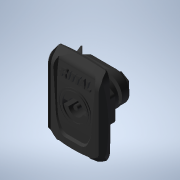
# Autodesk Inventor part: 1301.000_5_(1)
Saved by Autodesk Inventor 2021 (Build 250183000, 183)
## iProperties
Created: 2025-05-02
Part Number: 1301.000_5_(1)
Material: Generic
Catalog Web Link: www.cadenas.de
Description: Vorreibeverschluss EB Edelstahl 2.0-Vorreibeverschluss EB Edelstahl 2.0
Vendor: RITTAL
Document SubType Name: Modeling
Designer: psAdmin
Manufacturer: RITTAL
Mass: 18.9743 g
Surface Area: 89.9901 cm^2
Volume: 18.9743 cm^3
Density: 1 g/cm^3
Appearance: PSOLRGB-175-175-175
Category: PARTsolutions
Company: RITTAL
Title: 1301.000_5
Author: Cadenas PARTsolutions
Comments: Vorreibeverschluss EB Edelstahl 2.0
PSOL_IDENT_0: {$CADENAS_DATA/23d-libs/rittal/schaltschranksys/edelstahl/kleingehause/parts_eb_edel_2_0/vorreibever
PSOL_IDENT_1: schluss_kx_eb_edel_new.prj},205 {VTYP=3D},{NB=1301.000_5_(1)},{LINA=1301.000_5},{NN=Vorreibeverschlu
PSOL_IDENT_2: ss EB Edelstahl 2.0},{DATE=28.04.2025 21:10:48},{GEOMDATE=11.04.2025 11:21:29},{VERSION=},{LINEID=80
PSOL_IDENT_3: },{WBVAR=DETAIL},{WBNUMERIC=DETAIL}  {NB=1301.000_5_(1)},{LINA=1301.000_5},{KT=DUMMY},{BEST=1301.000
PSOL_IDENT_4: },{DETAIL=1},{GEW=3,889},{VERS=2},{CNSETIM80=EC000261},{CNSETIM90=EC000261},{CNSECLASS60=27-18-01-01
PSOL_IDENT_5: },{CNSECLASS80=27-18-01-01},{UNSPSC=31-26-15-02}
NB: 1301.000_5_(1)
NN: Vorreibeverschluss EB Edelstahl 2.0
NT: Vorreibeverschluss EB Edelstahl 2.0
NBSYN: $BEST._5_($DETAIL.)
LINA: 1301.000_5
CATALOG: Rittal
BEST: 1301.000
DETAIL: hoch
GEW: 3,889
VERS: 2
CNSETIM80: EC000261
CNSETIM90: EC000261
CNSECLASS60: 27-18-01-01
CNSECLASS80: 27-18-01-01
UNSPSC: 31-26-15-02
SUPPLIER: RITTAL
ARTICLENO: 1301.000_5_(1)
BOMINFO: 1301.000_5
CREATOR: CADENAS GmbH
Autodesk Inventor part; units mm, degrees
ref_plane "YZ Plane" through (0, 0, 0) normal (1, 0, 0) x (0, 1, 0)
ref_plane "XZ Plane" through (0, 0, 0) normal (0, 1, 0) x (-1, 0, 0)
ref_plane "XY Plane" through (0, 0, 0) normal (0, 0, 1) x (1, 0, 0)
sketch "Sketch_6" plane through (0, 0, 0) normal (0, -1, 0) x (1, 0, 0)
  line L0 (-17.65, 1.3) -> (-17.65, 0)
  line L1 (-17.65, 0) -> (17.65, 0)
  line L2 (17.65, 0) -> (17.65, 1.3)
  line L3 (17.65, 1.3) -> (16.6449, 7)
  line L4 (16.6449, 7) -> (-16.6449, 7)
  line L5 (-16.6449, 7) -> (-17.65, 1.3)
  constraints: 12 end point
extrude "Extrusion1" add sketch "Sketch_6" along normal mid plane 55.1
sketch "Sketch_1" plane through (0, 0, 7) normal (0, 0, 1) x (1, 0, 0)
  line L0 (-15.2906, 36.1) -> (-14.1918, 16.1075)
  arc A0 (-14.1918, 16.1075) -> (-14.0539, 14.1707) centre (45.7178, 19.4001) ccw
  line L1 (-14.0539, 14.1707) -> (-12.1282, -7.84)
  arc A1 (-12.1282, -7.84) -> (-10.69, -13.2074) centre (3.8109, -6.4455) ccw
  line L2 (-10.69, -13.2074) -> (-9.7308, -15.2644)
  arc A2 (-9.7308, -15.2644) -> (-4.7461, -18.44) centre (-4.7461, -12.94) ccw
  line L3 (-4.7461, -18.44) -> (4.7461, -18.44)
  arc A3 (4.7461, -18.44) -> (9.7308, -15.2644) centre (4.7461, -12.94) ccw
  line L4 (9.7308, -15.2644) -> (10.69, -13.2074)
  arc A4 (10.69, -13.2074) -> (12.1282, -7.84) centre (-3.8109, -6.4455) ccw
  line L5 (12.1282, -7.84) -> (14.0539, 14.1707)
  arc A5 (14.0539, 14.1707) -> (14.1918, 16.1075) centre (-45.7178, 19.4001) ccw
  line L6 (14.1918, 16.1075) -> (15.2906, 36.1)
  line L7 (15.2906, 36.1) -> (-15.2906, 36.1)
  constraints: 16 end point, 12 point on circle, 6 centre point
extrude "Extrusion2" cut sketch "Sketch_1" against normal blind 5.7 draft -42
sketch "Sketch_43" plane through (0, 0, 0) normal (0, 0, 1) x (1, 0, 0)
  line L0 (-10.3, 19.67) -> (-10.3, 13.67)
  line L1 (-10.3, 13.67) -> (10.6, 13.67)
  line L2 (10.6, 13.67) -> (10.6, 19.67)
  line L3 (10.6, 19.67) -> (-10.3, 19.67)
  constraints: 8 end point
extrude "Extrusion3" add sketch "Sketch_43" along normal blind 6
sketch "Sketch_44" plane through (0, 0, 6) normal (0, 0, 1) x (1, 0, 0)
  line L0 (-10.3, 19.67) -> (-10.3, 13.67)
  line L1 (-10.3, 13.67) -> (10.6, 13.67)
  line L2 (10.6, 13.67) -> (10.6, 19.67)
  line L3 (10.6, 19.67) -> (-10.3, 19.67)
  line L4 (6.723, 14.166) -> (10.118, 14.163)
  line L5 (10.118, 14.163) -> (10.118, 15.294)
  line L6 (10.118, 15.294) -> (8.245, 15.296)
  line L7 (8.245, 15.296) -> (9.308, 19.31)
  line L8 (9.308, 19.31) -> (8.088, 19.312)
  line L9 (8.088, 19.312) -> (6.723, 14.166)
  line L10 (1.861, 14.171) -> (3.212, 14.17)
  line L11 (3.212, 14.17) -> (3.783, 15.104)
  line L12 (3.783, 15.104) -> (5.252, 15.102)
  line L13 (5.252, 15.102) -> (5.324, 14.167)
  line L14 (5.324, 14.167) -> (6.584, 14.167)
  line L15 (6.584, 14.167) -> (6.063, 19.317)
  line L16 (6.063, 19.317) -> (5.132, 19.318)
  line L17 (5.132, 19.318) -> (1.861, 14.171)
  line L18 (0.388, 14.17) -> (1.615, 14.171)
  line L19 (1.615, 14.171) -> (2.697, 18.191)
  line L20 (2.697, 18.191) -> (3.434, 18.191)
  line L21 (3.434, 18.191) -> (3.738, 19.323)
  line L22 (3.738, 19.323) -> (0.875, 19.322)
  line L23 (0.875, 19.322) -> (0.57, 18.19)
  line L24 (0.57, 18.19) -> (1.472, 18.19)
  line L25 (1.472, 18.19) -> (0.388, 14.17)
  line L26 (-2.753, 14.17) -> (-1.526, 14.171)
  line L27 (-1.526, 14.171) -> (-0.444, 18.191)
  line L28 (-0.444, 18.191) -> (0.292, 18.191)
  line L29 (0.292, 18.191) -> (0.596, 19.323)
  line L30 (0.596, 19.323) -> (-2.267, 19.322)
  line L31 (-2.267, 19.322) -> (-2.571, 18.19)
  line L32 (-2.571, 18.19) -> (-1.669, 18.19)
  line L33 (-1.669, 18.19) -> (-2.753, 14.17)
  line L34 (-5.308, 14.168) -> (-4.083, 14.169)
  line L35 (-4.083, 14.169) -> (-2.693, 19.322)
  line L36 (-2.693, 19.322) -> (-3.916, 19.32)
  line L37 (-3.916, 19.32) -> (-5.308, 14.168)
  line L38 (-9.987, 17.217) -> (-9.987, 16.139)
  line L39 (-9.987, 16.139) -> (-9.151, 16.14)
  line L40 (-9.151, 16.14) -> (-9.687, 14.161)
  line L41 (-9.687, 14.161) -> (-8.467, 14.163)
  line L42 (-8.467, 14.163) -> (-7.936, 16.124)
  line L43 (-7.936, 16.124) -> (-7.443, 16.125)
  line L44 (-7.443, 16.125) -> (-6.993, 14.165)
  line L45 (-6.993, 14.165) -> (-5.649, 14.166)
  line L46 (-5.649, 14.166) -> (-6.179, 16.315)
  arc A0 (-6.179, 16.315) -> (-5.144, 17.102) centre (-6.971, 18.4306) ccw
  arc A1 (-5.144, 17.102) -> (-5.144, 18.833) centre (-6.4742, 17.9675) ccw
  arc A2 (-5.144, 18.833) -> (-6.3, 19.316) centre (-6.2287, 17.8617) ccw
  line L47 (-6.3, 19.316) -> (-8.293, 19.312)
  line L48 (-8.293, 19.312) -> (-8.86, 17.218)
  line L49 (-8.86, 17.218) -> (-9.987, 17.217)
  constraints: 100 end point, 6 point on circle, 3 centre point
extrude "Extrusion4" cut sketch "Sketch_44" against normal blind 2
sketch "Sketch_46" plane through (0, 0, 6) normal (0, 0, 1) x (1, 0, 0)
  line L0 (-7.614, 17.216) -> (-6.897, 17.216)
  arc A0 (-6.897, 17.216) -> (-6.428, 17.356) centre (-6.8725, 17.9896) ccw
  arc A1 (-6.428, 17.356) -> (-6.13, 17.839) centre (-6.9274, 17.9975) ccw
  arc A2 (-6.13, 17.839) -> (-6.192, 18.075) centre (-6.3798, 17.8995) ccw
  arc A3 (-6.192, 18.075) -> (-6.457, 18.174) centre (-6.4312, 17.839) ccw
  line L1 (-6.457, 18.174) -> (-7.356, 18.174)
  line L2 (-7.356, 18.174) -> (-7.614, 17.216)
  constraints: 8 point on circle, 6 end point, 4 centre point
extrude "Extrusion5" cut sketch "Sketch_46" against normal blind 2
sketch "Sketch_47" plane through (0, 0, 6) normal (0, 0, 1) x (1, 0, 0)
  line L0 (4.4417, 16.1815) -> (5.2647, 16.1805)
  line L1 (5.2647, 16.1805) -> (5.2027, 17.4445)
  line L2 (5.2027, 17.4445) -> (4.4417, 16.1815)
  constraints: 6 end point
extrude "Extrusion6" cut sketch "Sketch_47" against normal blind 2
sketch "Sketch_2" plane through (0, 0, 7) normal (1, 0, 0) x (0, 0, -1)
  arc A0 (2.6402, 21.4) -> (1.4014, -20) centre (279.4, -7.6) ccw
  arc A1 (1.4014, -20) -> (4.1718, -25.8207) centre (8.9014, -20) ccw
  line L0 (4.1718, -25.8207) -> (6.3, -27.55)
  line L1 (6.3, -27.55) -> (6.3, 27.55)
  line L2 (6.3, 27.55) -> (5.7, 27.55)
  line L3 (5.7, 27.55) -> (3.5376, 24.258)
  arc A2 (3.5376, 24.258) -> (2.6402, 21.4) centre (7.6402, 21.4) ccw
  constraints: 8 end point, 6 point on circle, 3 centre point
extrude "Extrusion7" add sketch "Sketch_2" along normal mid plane 32
sketch "Sketch_5" plane through (0, 0, 0) normal (0, 0, 1) x (1, 0, 0)
  line L0 (-40, -50) -> (40, -50)
  line L1 (40, -50) -> (40, 50)
  line L2 (40, 50) -> (-40, 50)
  line L3 (-40, 50) -> (-40, -50)
  arc A0 (-17.177, 19.885) -> (-17.448, -18.485) centre (559.8053, -3.3761) ccw
  arc A1 (-17.448, -18.485) -> (-17.092, -21.203) centre (-6.801, -18.4728) ccw
  arc A2 (-17.092, -21.203) -> (-16.213, -23.36) centre (-4.8797, -17.484) ccw
  arc A3 (-16.213, -23.36) -> (-15.393, -24.9) centre (8.4697, -11.2056) ccw
  arc A4 (-15.393, -24.9) -> (-12.239, -26.766) centre (4.8714, 5.7533) ccw
  arc A5 (-12.239, -26.766) -> (-12.0566, -26.7175) centre (-13.4109, -21.9938) ccw
  arc A6 (-12.0566, -26.7175) -> (12.0566, -26.7175) centre (0, 72) ccw
  arc A7 (12.0566, -26.7175) -> (12.239, -26.766) centre (13.4109, -21.9938) ccw
  arc A8 (12.239, -26.766) -> (15.393, -24.9) centre (-4.8714, 5.7533) ccw
  arc A9 (15.393, -24.9) -> (16.213, -23.36) centre (-8.4697, -11.2056) ccw
  arc A10 (16.213, -23.36) -> (17.092, -21.203) centre (4.8797, -17.484) ccw
  arc A11 (17.092, -21.203) -> (17.448, -18.485) centre (6.801, -18.4728) ccw
  arc A12 (17.448, -18.485) -> (17.177, 19.885) centre (-559.8053, -3.3761) ccw
  arc A13 (17.177, 19.885) -> (16.263, 24.293) centre (6.3822, 19.9454) ccw
  arc A14 (16.263, 24.293) -> (15.412, 26.294) centre (-21.6414, 9.3542) ccw
  line L4 (15.412, 26.294) -> (14.58, 26.682)
  line L5 (14.58, 26.682) -> (14.2616, 26.6294)
  arc A15 (14.2616, 26.6294) -> (-14.2616, 26.6294) centre (0, -75.227) ccw
  line L6 (-14.2616, 26.6294) -> (-14.58, 26.682)
  line L7 (-14.58, 26.682) -> (-15.412, 26.294)
  arc A16 (-15.412, 26.294) -> (-16.263, 24.293) centre (21.6414, 9.3542) ccw
  arc A17 (-16.263, 24.293) -> (-17.177, 19.885) centre (-6.3822, 19.9454) ccw
  constraints: 36 point on circle, 18 centre point, 16 end point
extrude "Extrusion8" cut sketch "Sketch_5" along normal blind 20
sketch "Sketch_7" plane through (0, 27.55, 1.3) normal (0, -0.7660444, 0.6427876) x (1, 0, 0)
  line L0 (-38, -25) -> (-17.65, -25)
  line L1 (-17.65, -25) -> (-17.65, -1.5387)
  line L2 (-17.65, -1.5387) -> (-16.8432, -0.3865)
  arc A0 (-16.3432, -0.3049) -> (-16.8432, -0.3865) centre (0, -102) ccw
  line L3 (-16.3432, -0.3049) -> (-15.593, -1.1989)
  arc A1 (15.593, -1.1989) -> (-15.593, -1.1989) centre (0, -102) ccw
  line L4 (15.593, -1.1989) -> (16.3432, -0.3049)
  arc A2 (16.8432, -0.3865) -> (16.3432, -0.3049) centre (0, -102) ccw
  line L5 (16.8432, -0.3865) -> (17.65, -1.5387)
  line L6 (17.65, -1.5387) -> (17.65, -25)
  line L7 (17.65, -25) -> (35, -25)
  line L8 (35, -25) -> (35, 19)
  line L9 (35, 19) -> (-38, 19)
  line L10 (-38, 19) -> (-38, -25)
  constraints: 22 end point, 6 point on circle, 3 centre point
extrude "Extrusion9" cut sketch "Sketch_7" along normal blind 20
sketch "Sketch_8" plane through (0, 23.3368, 4.8353) normal (0, -0.7660444, 0.6427876) x (1, 0, 0)
  line L0 (50, -10) -> (-50, -10)
  line L1 (-38, -6) -> (-17.65, -6)
  line L2 (-17.65, -6) -> (-17.65, -1.5387)
  line L3 (-17.65, -1.5387) -> (-16.8432, -0.3865)
  arc A0 (-16.3432, -0.3049) -> (-16.8432, -0.3865) centre (0, -102) ccw
  line L4 (-16.3432, -0.3049) -> (-15.593, -1.1989)
  arc A1 (15.593, -1.1989) -> (-15.593, -1.1989) centre (0, -102) ccw
  line L5 (15.593, -1.1989) -> (16.3432, -0.3049)
  arc A2 (16.8432, -0.3865) -> (16.3432, -0.3049) centre (0, -102) ccw
  line L6 (16.8432, -0.3865) -> (17.65, -1.5387)
  line L7 (17.65, -1.5387) -> (17.65, -6)
  line L8 (17.65, -6) -> (35, -6)
  line L9 (35, -6) -> (35, 19)
  line L10 (35, 19) -> (-38, 19)
  line L11 (-38, 19) -> (-38, -6)
  constraints: 24 end point, 6 point on circle, 3 centre point
revolve "Revolution1" cut sketch "Sketch_8" angle 40 about axis through (50, 16.9089, -2.8251) along (1, 0, 0)
sketch "Sketch_9" plane through (0, 16.9089, 7.1749) normal (0, -1, 0) x (1, 0, 0)
  line L0 (-38, -6) -> (-17.65, -6)
  line L1 (-17.65, -6) -> (-17.65, -1.5387)
  line L2 (-17.65, -1.5387) -> (-16.8432, -0.3865)
  arc A0 (-16.3432, -0.3049) -> (-16.8432, -0.3865) centre (0, -102) ccw
  line L3 (-16.3432, -0.3049) -> (-15.593, -1.1989)
  arc A1 (15.593, -1.1989) -> (-15.593, -1.1989) centre (0, -102) ccw
  line L4 (15.593, -1.1989) -> (16.3432, -0.3049)
  arc A2 (16.8432, -0.3865) -> (16.3432, -0.3049) centre (0, -102) ccw
  line L5 (16.8432, -0.3865) -> (17.65, -1.5387)
  line L6 (17.65, -1.5387) -> (17.65, -6)
  line L7 (17.65, -6) -> (35, -6)
  line L8 (35, -6) -> (35, 19)
  line L9 (35, 19) -> (-38, 19)
  line L10 (-38, 19) -> (-38, -6)
  constraints: 22 end point, 6 point on circle, 3 centre point
extrude "Extrusion10" cut sketch "Sketch_9" along normal blind 43
sketch "Sketch_11" plane through (0, -27.55, 1.3) normal (0, 0.6427876, 0.7660444) x (1, 0, 0)
  line L0 (-41.5728, -20.604) -> (38.4272, -20.604)
  line L1 (38.4272, -20.604) -> (38.4272, 19.396)
  line L2 (38.4272, 19.396) -> (17.65, 19.396)
  line L3 (17.65, 19.396) -> (17.65, 4.3312)
  arc A0 (11.0304, 0.25) -> (17.65, 4.3312) centre (0, 25.55) ccw
  line L4 (11.0304, 0.25) -> (10.2426, 0.5367)
  arc A1 (-10.2426, 0.5367) -> (10.2426, 0.5367) centre (0, 98) ccw
  line L5 (-10.2426, 0.5367) -> (-11.0304, 0.25)
  arc A2 (-17.65, 4.3312) -> (-11.0304, 0.25) centre (0, 25.55) ccw
  line L6 (-17.65, 4.3312) -> (-17.65, 19.396)
  line L7 (-17.65, 19.396) -> (-41.5728, 19.396)
  line L8 (-41.5728, 19.396) -> (-41.5728, -20.604)
  constraints: 18 end point, 6 point on circle, 3 centre point
extrude "Extrusion11" cut sketch "Sketch_11" along normal blind 40
sketch "Sketch_17" plane through (0, 0, 0) normal (0, 1, 0) x (-1, 0, 0)
  line L0 (0, 0) -> (0, -21.4)
  line L1 (0, -19.9) -> (-6.95, -19.9)
  arc A0 (-6.95, -19.9) -> (-7.25, -20.2) centre (-6.95, -20.2) ccw
  line L2 (-7.25, -20.2) -> (-7.25, -20.6)
  arc A1 (-8.05, -21.4) -> (-7.25, -20.6) centre (-8.05, -20.6) ccw
  line L3 (-8.05, -21.4) -> (-8.5, -21.4)
  arc A2 (-9.5, -20.4) -> (-8.5, -21.4) centre (-8.5, -20.4) ccw
  line L4 (-9.5, -20.4) -> (-9.5, -15.9)
  line L5 (-9.5, -15.9) -> (-4.95, -15.9)
  line L6 (-4.95, -15.9) -> (-4.95, -15.8)
  line L7 (-4.95, -15.8) -> (-9.75, -15.8)
  line L8 (-9.75, -15.8) -> (-9.75, -9.7)
  line L9 (-9.75, -9.7) -> (-9.773, -9.7)
  line L10 (-9.773, -9.7) -> (-11, -8.473)
  line L11 (-11, -8.473) -> (-11, -2.5)
  line L12 (-11, -2.5) -> (-10.125, -2.5)
  line L13 (-10.125, -2.5) -> (-10.125, 0)
  line L14 (-10.125, 0) -> (0, 0)
  line L15 (0, 0) -> (0, -19.9)
  constraints: 32 end point, 6 point on circle, 3 centre point
revolve "Revolution2" add sketch "Sketch_17" angle 360 about axis through (0, 0, 0) along (0, 0, 1)
thread "Thread1" size "M22x2" class "6g" standard "ISO Metric profile" full length
sketch "Sketch_19" plane through (0, 0, 0) normal (0, 0, 1) x (1, 0, 0)
  line L0 (-11.1, 11.1) -> (-11.1, -11.1)
  line L1 (-11.1, -11.1) -> (11.1, -11.1)
  line L2 (11.1, -11.1) -> (11.1, 11.1)
  line L3 (11.1, 11.1) -> (-11.1, 11.1)
  line L4 (-10, -10) -> (10, -10)
  line L5 (10, -10) -> (10, 10)
  line L6 (10, 10) -> (-10, 10)
  line L7 (-10, 10) -> (-10, -10)
  constraints: 16 end point
extrude "Extrusion12" cut sketch "Sketch_19" against normal blind 10
sketch "Sketch_20" plane through (0, 0, 0) normal (0, 0, 1) x (1, 0, 0)
  arc A0 (-14.7, -10.2) -> (-10.2, -14.7) centre (-10.2, -10.2) ccw
  line L0 (-10.2, -14.7) -> (10.2, -14.7)
  arc A1 (10.2, -14.7) -> (14.7, -10.2) centre (10.2, -10.2) ccw
  line L1 (14.7, -10.2) -> (14.7, 10.2)
  arc A2 (14.7, 10.2) -> (10.2, 14.7) centre (10.2, 10.2) ccw
  line L2 (10.2, 14.7) -> (-10.2, 14.7)
  arc A3 (-10.2, 14.7) -> (-14.7, 10.2) centre (-10.2, 10.2) ccw
  line L3 (-14.7, 10.2) -> (-14.7, -10.2)
  constraints: 8 end point, 8 point on circle, 4 centre point
extrude "Extrusion13" add sketch "Sketch_20" against normal blind 1.07
sketch "Sketch_18" plane through (0, 0, -15.9) normal (0, 0, 1) x (1, 0, 0)
  line L0 (-10, 10.2) -> (-10, -2.8)
  line L1 (-10, -2.8) -> (-4.082, -2.8)
  arc A0 (4.082, -2.8) -> (-4.082, -2.8) centre (0, 0) ccw
  line L2 (4.082, -2.8) -> (10, -2.8)
  line L3 (10, -2.8) -> (10, 10.2)
  line L4 (10, 10.2) -> (-10, 10.2)
  constraints: 10 end point, 2 point on circle, 1 centre point
extrude "Extrusion14" cut sketch "Sketch_18" along normal blind 2.4
sketch "Sketch_21" plane through (0, 0, -15.9) normal (0, 0, 1) x (1, 0, 0)
  arc A0 (-5.5, 7.7942) -> (-5.5, -7.7942) centre (-1, 0) ccw
  line L0 (-5.5, -7.7942) -> (-4.75, -8.2272)
  arc A1 (-4.75, -8.2272) -> (-4.75, 8.2272) centre (0, 0) ccw
  line L1 (-4.75, 8.2272) -> (-5.5, 7.7942)
  constraints: 4 end point, 4 point on circle, 2 centre point
extrude "Extrusion15" add sketch "Sketch_21" against normal blind 4.5
sketch "Sketch_22" plane through (0, 0, -15.9) normal (0, 0, 1) x (1, 0, 0)
  arc A0 (-9.5534, 2.8) -> (-9.5534, -2.8) centre (-1, 0) ccw
  line L0 (-9.5534, -2.8) -> (0, -2.8)
  line L1 (0, -2.8) -> (0, 2.8)
  line L2 (0, 2.8) -> (-9.5534, 2.8)
  constraints: 6 end point, 2 point on circle, 1 centre point
extrude "Extrusion16" add sketch "Sketch_22" along normal blind 2.3
sketch "Sketch_23" plane through (0, 0, 0) normal (1, 0, 0) x (0, 1, 0)
  line L0 (6.5, -17.4) -> (-6.5, -17.4)
  line L1 (-6.5, -17.4) -> (-9.5, -18.7989)
  line L2 (-9.5, -18.7989) -> (-9.5, -20.4)
  arc A0 (-9.5, -20.4) -> (-8.5, -21.4) centre (-8.5, -20.4) ccw
  line L3 (-8.5, -21.4) -> (8.5, -21.4)
  arc A1 (8.5, -21.4) -> (9.5, -20.4) centre (8.5, -20.4) ccw
  line L4 (9.5, -20.4) -> (9.5, -18.7989)
  line L5 (9.5, -18.7989) -> (6.5, -17.4)
  constraints: 12 end point, 4 point on circle, 2 centre point
extrude "Extrusion17" add sketch "Sketch_23" against normal blind 20
sketch "Sketch_45" plane through (0, 0, 0) normal (0, 1, 0) x (-1, 0, 0)
  line L0 (28.466, -23.355) -> (23.0968, -17.9858)
  arc A0 (23.0968, -17.9858) -> (21.6826, -17.4) centre (21.6826, -19.4) ccw
  line L1 (21.6826, -17.4) -> (14.511, -17.4)
  line L2 (14.511, -17.4) -> (14.511, -21.4)
  line L3 (14.511, -21.4) -> (16.7433, -21.4)
  arc A1 (18.1575, -21.9858) -> (16.7433, -21.4) centre (16.7433, -23.4) ccw
  line L4 (18.1575, -21.9858) -> (21.3575, -25.1857)
  arc A2 (21.3575, -25.1857) -> (21.8057, -25.4445) centre (22.0646, -24.4786) ccw
  line L5 (21.8057, -25.4445) -> (24.853, -26.261)
  arc A3 (24.853, -26.261) -> (25.8189, -26.0022) centre (25.1118, -25.2951) ccw
  line L6 (25.8189, -26.0022) -> (28.466, -23.355)
  constraints: 14 end point, 8 point on circle, 4 centre point
extrude "Extrusion18" add sketch "Sketch_45" along normal mid plane 13.7
sketch "Sketch_24" plane through (-20.3897, 0, -15.2787) normal (-0.7071068, 0, -0.7071068) x (-0.7071068, 0, 0.7071068)
  line L0 (-4.0663, -9.85) -> (5, -9.85)
  line L1 (5, -9.85) -> (5, 9.85)
  line L2 (5, 9.85) -> (-4.0663, 9.85)
  line L3 (-4.0663, 9.85) -> (0, 3)
  line L4 (0, 3) -> (0, -3)
  line L5 (0, -3) -> (-4.0663, -9.85)
  constraints: 12 end point
extrude "Extrusion19" cut sketch "Sketch_24" along normal blind 13
sketch "Sketch_25" plane through (-20.319, 0, -19.592) normal (-0.7071068, 0, 0.7071068) x (0.7071068, 0, 0.7071068)
  line L0 (-21.047, 9.5) -> (-21.047, -9.5)
  line L1 (-21.047, -9.5) -> (2.078, -9.5)
  line L2 (2.078, -9.5) -> (2.078, -3.7)
  arc A0 (2.078, -3.7) -> (0.378, -2) centre (0.378, -3.7) ccw
  line L3 (0.378, -2) -> (-12.922, -2)
  line L4 (-12.922, -2) -> (-12.922, 2)
  line L5 (-12.922, 2) -> (0.378, 2)
  arc A1 (0.378, 2) -> (2.078, 3.7) centre (0.378, 3.7) ccw
  line L6 (2.078, 3.7) -> (2.078, 9.5)
  line L7 (2.078, 9.5) -> (-21.047, 9.5)
  constraints: 16 end point, 4 point on circle, 2 centre point
extrude "Extrusion20" cut sketch "Sketch_25" against normal blind 5
sketch "Sketch_26" plane through (-20.319, 0, -19.592) normal (-0.7071068, 0, 0.7071068) x (0.7071068, 0, 0.7071068)
  line L0 (-12.922, -10.85) -> (2.078, -10.85)
  line L1 (2.078, -10.85) -> (2.078, -6.85)
  line L2 (2.078, -6.85) -> (-12.922, -6.85)
  line L3 (-12.922, -6.85) -> (-12.922, -10.85)
  constraints: 8 end point
extrude "Extrusion21" cut sketch "Sketch_26" along normal blind 3
sketch "Sketch_27" plane through (-20.319, 0, -19.592) normal (-0.7071068, 0, 0.7071068) x (0.7071068, 0, 0.7071068)
  line L0 (-12.922, 10.85) -> (-12.922, 6.85)
  line L1 (-12.922, 6.85) -> (2.078, 6.85)
  line L2 (2.078, 6.85) -> (2.078, 10.85)
  line L3 (2.078, 10.85) -> (-12.922, 10.85)
  constraints: 8 end point
extrude "Extrusion22" cut sketch "Sketch_27" along normal blind 3
sketch "Sketch_28" plane through (-22.511, 0, -17.4) normal (1, 0, 0) x (0, 0, -1)
  line L0 (-3, 9.5) -> (-3, -9.5)
  line L1 (-3, -9.5) -> (1.3989, -9.5)
  line L2 (1.3989, -9.5) -> (0, -6.5)
  line L3 (0, -6.5) -> (0, 6.5)
  line L4 (0, 6.5) -> (1.3989, 9.5)
  line L5 (1.3989, 9.5) -> (-3, 9.5)
  constraints: 12 end point
extrude "Extrusion23" cut sketch "Sketch_28" along normal blind 8
sketch "Sketch_36" plane through (0, 0, 0) normal (0, 1, 0) x (-1, 0, 0)
  line L0 (0, 0) -> (0, -21.4)
  line L1 (0, -21.4) -> (-8.05, -21.4)
  arc A0 (-8.05, -21.4) -> (-7.25, -20.6) centre (-8.05, -20.6) ccw
  line L2 (-7.25, -20.6) -> (-7.25, -20.2)
  arc A1 (-6.95, -19.9) -> (-7.25, -20.2) centre (-6.95, -20.2) ccw
  line L3 (-6.95, -19.9) -> (0, -19.9)
  line L4 (0, -19.9) -> (0, -21.4)
  constraints: 10 end point, 4 point on circle, 2 centre point
revolve "Revolution3" cut sketch "Sketch_36" angle 360 about axis through (0, 0, 0) along (0, 0, 1)
sketch "Sketch_10" plane through (0, 0, 0) normal (0, 0, 1) x (1, 0, 0)
  circle A0 centre (0, 0) radius 9.05
  constraints: 1 centre point
extrude "Extrusion24" add sketch "Sketch_10" along normal blind 6
sketch "Sketch_12" plane through (0, 0, 6) normal (0, 0, 1) x (1, 0, 0)
  circle A0 centre (0, 0) radius 8
  constraints: 1 centre point
extrude "Extrusion25" cut sketch "Sketch_12" along normal mid plane 1.4
sketch "Sketch_16" plane through (0, 0, 0) normal (0, 0, 1) x (1, 0, 0)
  circle A0 centre (0, 0) radius 10.75
  circle A1 centre (0, 0) radius 10
  constraints: 2 centre point
extrude "Extrusion26" add sketch "Sketch_16" along normal blind 6
sketch "Sketch_13" plane through (0, 0, 5.3) normal (0, 0, 1) x (1, 0, 0)
  arc A0 (-7.8581, 1.5) -> (-7.8581, -1.5) centre (0, 0) ccw
  line L0 (-7.8581, -1.5) -> (-4.7697, -1.5)
  arc A1 (-4.7697, -1.5) -> (4.7697, -1.5) centre (0, 0) ccw
  line L1 (4.7697, -1.5) -> (7.8581, -1.5)
  arc A2 (7.8581, -1.5) -> (7.8581, 1.5) centre (0, 0) ccw
  line L2 (7.8581, 1.5) -> (4.7697, 1.5)
  arc A3 (4.7697, 1.5) -> (-4.7697, 1.5) centre (0, 0) ccw
  line L3 (-4.7697, 1.5) -> (-7.8581, 1.5)
  circle A4 centre (0, 0) radius 1.5
  constraints: 8 end point, 8 point on circle, 5 centre point
extrude "Extrusion27" cut sketch "Sketch_13" against normal blind 7.5
sketch "Sketch_14" plane through (0, 0, -19.9) normal (0, 0, 1) x (1, 0, 0)
  line L0 (-5, -2.8868) -> (0, -5.7735)
  line L1 (0, -5.7735) -> (5, -2.8868)
  line L2 (5, -2.8868) -> (5, 2.8868)
  line L3 (5, 2.8868) -> (0, 5.7735)
  line L4 (0, 5.7735) -> (-5, 2.8868)
  line L5 (-5, 2.8868) -> (-5, -2.8868)
  constraints: 12 end point
extrude "Extrusion28" add sketch "Sketch_14" against normal blind 5
sketch "Sketch_35" plane through (0, 0, 0) normal (0, 1, 0) x (-1, 0, 0)
  line L0 (0, -19.9) -> (0, -20.15)
  arc A0 (-6.75, -20.1497) -> (0, -20.8997) centre (-1.423, -2.956) ccw
  line L1 (-6.75, -20.1497) -> (-6.75, -19.9)
  line L2 (-6.75, -19.9) -> (0, -19.9)
  line L3 (0, -19.9) -> (0, -20.8997)
  constraints: 8 end point, 2 point on circle, 1 centre point
revolve "Revolution4" add sketch "Sketch_35" angle 360 about axis through (0, 0, -19.9) along (0, 0, 1)
sketch "Sketch_40" plane through (0, 0, 0) normal (1, 0, 0) x (0, 1, 0)
  line L0 (0, -7.4) -> (0, -2.6)
  line L1 (11.5, -2.6) -> (10.3, -3.2928)
  line L2 (10.3, -3.2928) -> (10.3, -6.7072)
  line L3 (10.3, -6.7072) -> (11.5, -7.4)
  line L4 (11.5, -7.4) -> (15.3, -7.4)
  line L5 (15.3, -7.4) -> (15.3, -2.6)
  line L6 (15.3, -2.6) -> (11.5, -2.6)
  constraints: 14 end point
revolve "Revolution5" add sketch "Sketch_40" angle 360 about axis through (0, 0, -7.4) along (0, 0, -1)
sketch "Sketch_41" plane through (0, 0, -7.4) normal (0, 0, 1) x (1, 0, 0)
  line L0 (-27, -27) -> (27, -27)
  line L1 (27, -27) -> (27, 27)
  line L2 (27, 27) -> (-27, 27)
  line L3 (-27, 27) -> (-27, -27)
  arc A0 (-13.5, -6.6395) -> (-12.5, -8.3716) centre (-11.5, -6.6395) ccw
  line L4 (-12.5, -8.3716) -> (-1, -15.0111)
  arc A1 (-1, -15.0111) -> (1, -15.0111) centre (0, -13.2791) ccw
  line L5 (1, -15.0111) -> (12.5, -8.3716)
  arc A2 (12.5, -8.3716) -> (13.5, -6.6395) centre (11.5, -6.6395) ccw
  line L6 (13.5, -6.6395) -> (13.5, 6.6395)
  arc A3 (13.5, 6.6395) -> (12.5, 8.3716) centre (11.5, 6.6395) ccw
  line L7 (12.5, 8.3716) -> (1, 15.0111)
  arc A4 (1, 15.0111) -> (-1, 15.0111) centre (0, 13.2791) ccw
  line L8 (-1, 15.0111) -> (-12.5, 8.3716)
  arc A5 (-12.5, 8.3716) -> (-13.5, 6.6395) centre (-11.5, 6.6395) ccw
  line L9 (-13.5, 6.6395) -> (-13.5, -6.6395)
  constraints: 20 end point, 12 point on circle, 6 centre point
extrude "Extrusion29" cut sketch "Sketch_41" along normal blind 4.8
sketch "Sketch_29" plane through (0, 0, -2.6) normal (0, 0, 1) x (1, 0, 0)
  arc A0 (-13.5, -6.6395) -> (-12.5, -8.3716) centre (-11.5, -6.6395) ccw
  line L0 (-12.5, -8.3716) -> (-9.8827, -9.8827)
  line L1 (-9.8827, -9.8827) -> (-9.5459, -9.5459)
  arc A1 (-13.04, -3.4941) -> (-9.5459, -9.5459) centre (0, 0) ccw
  line L2 (-13.04, -3.4941) -> (-13.5, -3.6173)
  line L3 (-13.5, -3.6173) -> (-13.5, -6.6395)
  constraints: 8 end point, 4 point on circle, 2 centre point
extrude "Extrusion30" add sketch "Sketch_29" along normal blind 0.6
pattern_circular "Circular Pattern1" count 6 over 360 about axis through (0, 0, -2.6) along (0, 0, 1) of "Extrusion30"
sketch "Sketch_37" plane through (0, 0, 0) normal (1, 0, 0) x (0, 1, 0)
  line L0 (0, -2) -> (0, 2)
  line L1 (16.5, -1.5) -> (13.5, -1.5)
  line L2 (13.5, -1.5) -> (13.5, -2)
  line L3 (13.5, -2) -> (16.5, -3.3989)
  line L4 (16.5, -3.3989) -> (16.5, -1.5)
  constraints: 10 end point
revolve "Revolution6" cut sketch "Sketch_37" angle 360 about axis through (0, 0, -2) along (0, 0, -1)
ref_plane "VV_XY" through (0, 0, 0) normal (0, 0, 1) x (1, 0, 0)
ref_plane "VV_YZ" through (0, 0, 0) normal (1, 0, 0) x (0, 1, 0)
ref_plane "VV_ZX" through (0, 0, 0) normal (0, 1, 0) x (0, 0, 1)
body "Solid1"
